bottombase (Autodesk Fusion 360 design; units mm, degrees)
Autodesk Fusion 360 part; units mm, degrees
sketch "Sketch1" plane through (0, 0, 0) normal (0, 0, 1) x (1, 0, 0)
  circle A0 centre (0, 0) radius 50
  line L0 (7.5, -45) -> (-7.5, -45)
  line L1 (-7.5, -45) -> (-7.5, -10)
  line L2 (-7.5, -10) -> (7.5, -10)
  line L3 (7.5, -10) -> (7.5, -45)
  line L4 (7.5, -45) -> (-7.5, -10) construction
  line L5 (-7.5, -45) -> (7.5, -10) construction
  line L6 (7.5, -35) -> (-7.5, -35)
  line L7 (-7.5, -35) -> (-7.5, -20)
  line L8 (-7.5, -20) -> (7.5, -20)
  line L9 (7.5, -20) -> (7.5, -35)
  line L10 (7.5, -35) -> (-7.5, -20) construction
  line L11 (-7.5, -35) -> (7.5, -20) construction
  point P0 (0, -27.5)
  point P1 (0, -27.5)
  dimension "d1" = 100
  dimension "d2" = 15
  dimension "d3" = 35
  dimension "d4" = 10
  dimension "d5" = 15
  constraint coincident A0.centre origin
  constraint horizontal L0
  constraint perpendicular L0 L1
  constraint parallel L0 L2
  constraint parallel L1 L3
  constraint coincident L4 P1
  constraint coincident L5 P1
  constraint horizontal L6
  constraint perpendicular L6 L7
  constraint parallel L6 L8
  constraint parallel L7 L9
  constraint coincident L10 P1
  constraint coincident L11 P1
  constraint coincident P1 P0
  measures "d1" diameter of A0
  measures "d2" distance of L1.end L2.end
  measures "d3" distance of L0.end L1.end
  measures "d4" distance of A0.centre L2
  measures "d5" distance of L6.end L7.end
extrude "Extrude1" add sketch "Sketch1" along normal blind 10
sketch "Sketch2" plane through (0, 0, 0) normal (0, 1, 0) x (1, 0, 0)
  line L0 (-7.5, 0, -45) -> (7.5, 0, -45)
  line L1 (7.5, 0, -45) -> (7.5, -40, -45)
  line L2 (7.5, -40, -45) -> (-7.5, -40, -45)
  line L3 (-7.5, -40, -45) -> (-7.5, 0, -45)
  circle A0 through (7.5, -32.5, -45) (-3.75, -26.0048, -45) (-3.75, -38.9952, -45)
  circle A1 through (3.75, -32.5, -45) (-1.875, -29.2524, -45) (-1.875, -35.7476, -45)
  line L4 (-7.5, 0, -45) -> (7.5, 0, -45)
  line L5 (7.5, 0, -45) -> (7.5, -25, -45)
  line L6 (7.5, -25, -45) -> (-7.5, -25, -45)
  line L7 (-7.5, -25, -45) -> (-7.5, 0, -45)
  dimension "d8" = 15
  dimension "d9" = 40
  dimension "d10" = 7.5
  dimension "d11" = 25
sketch "Sketch2 (curves -45 mm off its plane)" plane through (0, -45, 0) normal (0, 1, 0) x (1, 0, 0)
  line L0 (-7.5, 0) -> (7.5, 0)
  line L1 (7.5, 0) -> (7.5, -40)
  line L2 (7.5, -40) -> (-7.5, -40)
  line L3 (-7.5, -40) -> (-7.5, 0)
  circle A0 centre (0, -32.5) radius 7.5
  circle A1 centre (0, -32.5) radius 3.75
  line L4 (-7.5, 0) -> (7.5, 0)
  line L5 (7.5, 0) -> (7.5, -25)
  line L6 (7.5, -25) -> (-7.5, -25)
  line L7 (-7.5, -25) -> (-7.5, 0)
extrude "Extrude2" add sketch "Sketch2 (curves -45 mm off its plane)" along normal blind 35 contours L0 L1 L3 L4 L5 L6 L7 | L3 A0 L6 | L1 A0 L6 | A0
extrude "Extrude3" cut sketch "Sketch1" along normal blind 40 contours L1 L3 L6 L7 L8 L9
extrude "Extrude4" add sketch "Sketch1" along normal blind 25 contours L1 L3 L6 L7 L8 L9
pattern_circular "C-Pattern1" count 3 over 360 about axis through (0, 0, 1.75) along (0, 0, 1) of "Extrude2", "Extrude3", "Extrude4"
sketch "Sketch3" plane through (0, 0, 10) normal (0, 0, 1) x (-1, 0, 0)
  line L0 (12.4103, 1.4952) -> (42.7211, -16.0048)
  line L1 (42.7211, -16.0048) -> (35.2211, -28.9952)
  line L2 (35.2211, -28.9952) -> (4.9103, -11.4952)
  line L3 (4.9103, -11.4952) -> (12.4103, 1.4952)
  line L4 (-4.9103, -11.4952) -> (-35.2211, -28.9952)
  line L5 (-35.2211, -28.9952) -> (-42.7211, -16.0048)
  line L6 (-42.7211, -16.0048) -> (-12.4103, 1.4952)
  line L7 (-12.4103, 1.4952) -> (-4.9103, -11.4952)
  line L8 (-7.5, 10) -> (-7.5, 45)
  line L9 (-7.5, 45) -> (7.5, 45)
  line L10 (7.5, 45) -> (7.5, 10)
  line L11 (7.5, 10) -> (-7.5, 10)
  circle A0 centre (0, 0) radius 50
  line L12 (-11.547, 20) -> (-23.094, 0)
  line L13 (-23.094, 0) -> (-11.547, -20)
  line L14 (-11.547, -20) -> (11.547, -20)
  line L15 (11.547, -20) -> (23.094, 0)
  line L16 (23.094, 0) -> (11.547, 20)
  line L17 (11.547, 20) -> (-11.547, 20)
  constraint coincident A0.centre origin
extrude "Extrude5" add sketch "Sketch3" along normal blind 15 contours L0 L2 L3 L4 L6 L7 L8 L10 L11 L12 L13 L14 L15 L16 L17
equation "d10 = ( 15 / 2 ) * 1 mm"
